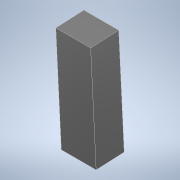
# Autodesk Inventor part: battery
Saved by Autodesk Inventor 2022 (Build 260153070, 153G)
## iProperties
Created: 2021-05-24
Part Number: battery
Material: ABS Plastic
Document SubType Name: Modeling
Designer: kardo
Density: 1.06 g/cm^3
Appearance: Smooth - White
Mass: 220 g
Surface Area: 166.48 cm^2
Volume: 116.928 cm^3
Author: kardo
Autodesk Inventor part; units mm, degrees
ref_plane "YZ Plane" through (0, 0, 0) normal (1, 0, 0) x (0, 1, 0)
ref_plane "XZ Plane" through (0, 0, 0) normal (0, 1, 0) x (-1, 0, 0)
ref_plane "XY Plane" through (0, 0, 0) normal (0, 0, 1) x (1, 0, 0)
derived "powertrain_outline.ipt"
sketch "sk_electronics" plane through (6.24, 0, 0) normal (1, 0, 0) x (0, 1, 0)
  line L0 (-84.4095, 51.3017) -> (-84.7665, 21.3038)
  line L1 (-84.7665, 21.3038) -> (-44.7693, 20.8279)
  line L2 (-44.7693, 20.8279) -> (-44.4123, 50.8258)
  line L3 (-44.4123, 50.8258) -> (-84.4095, 51.3017)
  line L4 (-84.4095, 51.3017) -> (-44.7693, 20.8279) construction
  line L5 (-84.7665, 21.3038) -> (-44.4123, 50.8258) construction
  line L6 (-37.363, 49.7305) -> (-35.8962, 20.7676)
  line L7 (-35.8962, 20.7676) -> (75.9605, 26.4327)
  line L8 (75.9605, 26.4327) -> (74.4936, 55.3956)
  line L9 (74.4936, 55.3956) -> (-37.363, 49.7305)
  line L10 (-37.363, 49.7305) -> (75.9605, 26.4327) construction
  line L11 (-35.8962, 20.7676) -> (74.4936, 55.3956) construction
  line L12 (-84.7665, 21.3038) -> (-84.7665, 18.3038) construction
  line L13 (-44.7693, 20.8279) -> (-44.7693, 17.8279) construction
  line L14 (-35.8962, 20.7676) -> (-35.8962, 17.7676) construction
  line L15 (75.9605, 26.4327) -> (75.9605, 23.4327) construction
  spline S0 degree 4 poles (-297.6664, 19.4083) (-178.2238, 21.0761) (-46.6271, 18.3209) (53.0846, 11.363) (94.8, 28.832) knots 0 0 0 0 0 1 1 1 1 1
  point P0 (0, 0)
  point P1 (-64.5894, 36.0648)
  point P2 (19.2987, 38.0816)
sketch "Sketch2" plane through (0, 0, 0) normal (1, 0, 0) x (0, 1, 0)
  line L0 (74.4936, 55.3956) -> (-37.363, 49.7305) projected
  line L1 (75.9605, 26.4327) -> (74.4936, 55.3956) projected
  line L2 (-35.8962, 20.7676) -> (75.9605, 26.4327) projected
  line L3 (-37.363, 49.7305) -> (-35.8962, 20.7676) projected
  point P0 (0, 0)
extrude "Extrusion2" add sketch "Sketch2" along normal mid plane 36
body "Solid2"
